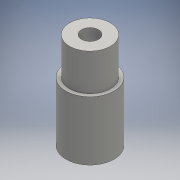
# Autodesk Inventor part: ピニオンギア 歯数8
Saved by Autodesk Inventor 2016 (Build 200138000, 138)
## iProperties
Created: 2018-12-09
Part Number: ピニオンギア 歯数8
Material: 一般
Document SubType Name: Modeling
Designer: mozar
Mass: 5 g
Surface Area: 4.01747 cm^2
Volume: 0.330244 cm^3
Density: 15.1403 g/cm^3
Appearance: 既定
Author: mozar
Autodesk Inventor part; units mm, degrees
ref_plane "YZ Plane" through (0, 0, 0) normal (1, 0, 0) x (0, 1, 0)
ref_plane "XZ Plane" through (0, 0, 0) normal (0, 1, 0) x (-1, 0, 0)
ref_plane "XY Plane" through (0, 0, 0) normal (0, 0, 1) x (1, 0, 0)
sketch "スケッチ1" plane through (0, 0, 0) normal (0, 0, 1) x (1, 0, 0)
  circle A0 centre (0, 0) radius 1.15
  circle A1 centre (0, 0) radius 3.25
  circle A2 centre (0, 0) radius 2.75
  dimension "d0" = 2.3
  dimension "d1" = 6.5
  dimension "d2" = 5.5
  constraints: 3 centre point, 3 coincident
  measures "d0" diameter of A0
  measures "d1" diameter of A1
  measures "d2" diameter of A2
extrude "押し出し1" add sketch "スケッチ1" along normal blind 5 contours A2
extrude "押し出し2" add sketch "スケッチ1" against normal blind 8 contours A1 | A2
